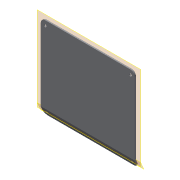
# Autodesk Inventor part: 03_Lid
Saved by Autodesk Inventor 2019.4 (Build 234330000, 330)
## iProperties
Created: 2021-06-05
Part Number: 03_Lid
Material: Generic
Document SubType Name: Modeling
Designer: diederichbenedict
Density: 1 g/cm^3
Appearance: Default
Author: diederichbenedict
Autodesk Inventor part; units mm, degrees
ref_plane "YZ Plane" through (0, 0, 0) normal (1, 0, 0) x (0, 1, 0)
ref_plane "XZ Plane" through (0, 0, 0) normal (0, 1, 0) x (-1, 0, 0)
ref_plane "XY Plane" through (0, 0, 0) normal (0, 0, 1) x (1, 0, 0)
ref_plane "Work Plane1" through (0, 0, 0) normal (0, 0, 1) x (1, 0, 0)
sketch "Sketch1" plane through (0, 0, 0) normal (0, 0, 1) x (1, 0, 0)
  ellipse E0 centre (-7.5, -84.2405) end of major axis (-7.5, -80.461) minor radius 1.5 projected
  ellipse E1 centre (-100.5, -84.2405) end of major axis (-100.5, -80.461) minor radius 1.5 projected
  ellipse E2 centre (-103, -7.7709) end of major axis (-103, -9.3506) minor radius 1.45 projected
  line L0 (-3, -61.2439) -> (-3, -12.7635) projected
  line L1 (-3, -61.2439) -> (-18, -61.2439) projected
  line L2 (-18, -90.5398) -> (-18, -61.2439) projected
  line L3 (0, -90.5398) -> (-18, -90.5398) projected
  line L4 (0, -7.7709) -> (0, -90.5398) projected
  ellipse E3 centre (-5, -7.7709) end of major axis (-5, -13.2183) minor radius 5 (0, -7.7709) -> (-5, -2.3235) ccw projected
  line L5 (-103, -2.3235) -> (-5, -2.3235) projected
  ellipse E4 centre (-103, -7.7709) end of major axis (-103, -13.2183) minor radius 5 (-103, -2.3235) -> (-108, -7.7709) ccw projected
  line L6 (-108, -90.5398) -> (-108, -7.7709) projected
  line L7 (-95, -90.5398) -> (-108, -90.5398) projected
  line L8 (-95, -61.2439) -> (-95, -90.5398) projected
  line L9 (-105, -61.2439) -> (-95, -61.2439) projected
  line L10 (-105, -12.7635) -> (-105, -61.2439) projected
  ellipse E5 centre (-103, -7.7709) end of major axis (-103, -13.2183) minor radius 5 (-105, -12.7635) -> (-98.4174, -5.5919) ccw projected
  line L11 (-9.5826, -5.5919) -> (-98.4174, -5.5919) projected
  ellipse E6 centre (-5, -7.7709) end of major axis (-5, -13.2183) minor radius 5 (-9.5826, -5.5919) -> (-3, -12.7635) ccw projected
  ellipse E7 centre (-5, -7.7709) end of major axis (-5, -9.3506) minor radius 1.45 projected
  line L12 (-18, -90.5398) -> (-95, -90.5398)
  point P0 (0, 0)
  constraints: 2 end point, 1 horizontal, 8 other
extrude "Extrusion1" add sketch "Sketch1" along normal blind 1.5 contours E0 | E1 | L1 L2 L12 L8 L9 L10 E5 L11 E6 L0 | L0 E6 L11 E5 L10 L9 L8 L7 L6 E4 L5 E3 L4 L3 L2 L1
ref_plane "Work Plane2" through (-54, -57.5226, 14.2761) normal (0, -0.3968725, 0.9178738) x (1, 0, 0)
sketch "Sketch2" plane through (-54, -57.5226, 14.2761) normal (0, -0.3968725, 0.9178738) x (1, 0, 0)
  circle A0 centre (49, -40) radius 1.45 projected
  circle A1 centre (-49, -40) radius 1.45 projected
  line L0 (-41, -35.9714) -> (-54, -35.9714) projected
  line L1 (-54, -40) -> (-54, -35.9714) projected
  arc A2 (-54, -40) -> (-49, -45) centre (-49, -40) ccw projected
  line L2 (49, -45) -> (-49, -45) projected
  arc A3 (49, -45) -> (54, -40) centre (49, -40) ccw projected
  line L3 (54, -35.9714) -> (54, -40) projected
  line L4 (54, -35.9714) -> (36, -35.9714) projected
  line L5 (36, -42) -> (36, -35.9714) projected
  line L6 (-41, -42) -> (36, -42) projected
  line L7 (-41, -35.9714) -> (-41, -42) projected
  line L8 (36, -35.9714) -> (-41, -35.9714)
  line L9 (-54, -35.9714) -> (54, -35.9714) projected
  line L10 (-54, 40) -> (-54, -35.9714) projected
  line L11 (54, -35.3761) -> (54, 40.5953) projected
  line L12 (-54, -35.9714) -> (54, -35.9714)
  line L13 (54, -35.9714) -> (54, -35.3761)
  line L14 (54, -35.3761) -> (-54, -35.3761)
  line L15 (-54, -35.3761) -> (-54, -35.9714)
  point P0 (54, 47.1327)
  constraints: 10 end point, 2 parallel, 1 collinear, 1 horizontal, 1 perpendicular
extrude "Extrusion2" add sketch "Sketch2" along normal up to surface (1.3768 mm away)
sketch "Sketch3" plane through (0, 0, 1.5) normal (0, 0, 1) x (1, 0, 0)
  ellipse E0 centre (-5, -7.7709) end of major axis (-5, -6.1911) minor radius 1.45 projected
  ellipse E1 centre (-103, -7.7709) end of major axis (-103, -6.1911) minor radius 1.45 projected
  line L0 (-108, -90.5398) -> (0, -90.5398) projected
  line L1 (0, -90.5398) -> (0, -7.7709) projected
  ellipse E2 centre (-5, -7.7709) end of major axis (-5, -13.2183) minor radius 5 (0, -7.7709) -> (-5, -2.3235) ccw projected
  line L2 (-5, -2.3235) -> (-103, -2.3235) projected
  ellipse E3 centre (-103, -7.7709) end of major axis (-103, -13.2183) minor radius 5 (-103, -2.3235) -> (-108, -7.7709) ccw projected
  line L3 (-108, -7.7709) -> (-108, -90.5398) projected
  line L4 (-3.7152, -59.4836) -> (-104.3916, -59.4836) construction
  line L5 (-104.3916, -59.4836) -> (-104.3916, -42.5544) construction
  line L6 (-104.3916, -42.5544) -> (-3.7152, -42.5544) construction
  line L7 (-3.7152, -42.5544) -> (-3.7152, -59.4836) construction
  spline S0 degree 2 poles (-14.2682, -57.7177) (-15.0084, -56.8506) (-15.8332, -54.3128) (-15.8332, -52.6844) knots 0 0 0 1 2 2 2
  spline S1 degree 2 poles (-15.8332, -52.6844) (-15.8332, -51.0983) (-15.0296, -48.5288) (-14.2682, -47.6617) knots 0 0 0 1 2 2 2
  spline S2 degree 2 poles (-14.2682, -47.6617) (-13.4646, -46.7523) (-11.3392, -45.8852) (-10.0597, -45.8852) knots 0 0 0 1 2 2 2
  spline S3 degree 2 poles (-10.0597, -45.8852) (-8.7379, -45.8852) (-6.6231, -46.784) (-5.8512, -47.6617) knots 0 0 0 1 2 2 2
  spline S4 degree 2 poles (-5.8512, -47.6617) (-5.1004, -48.5288) (-4.2968, -51.0771) (-4.2968, -52.6844) knots 0 0 0 1 2 2 2
  spline S5 degree 2 poles (-4.2968, -52.6844) (-4.2968, -54.3234) (-5.111, -56.8189) (-5.8618, -57.7177) knots 0 0 0 1 2 2 2
  spline S6 degree 2 poles (-5.8618, -57.7177) (-6.6231, -58.5848) (-8.7485, -59.4836) (-10.0597, -59.4836) knots 0 0 0 1 2 2 2
  spline S7 degree 2 poles (-10.0597, -59.4836) (-11.392, -59.4836) (-13.528, -58.553) (-14.2682, -57.7177) knots 0 0 0 1 2 2 2
  spline S8 degree 2 poles (-14.025, -52.6844) (-14.025, -53.9744) (-13.4646, -55.9729) (-12.957, -56.6285) knots 0 0 0 1 2 2 2
  spline S9 degree 2 poles (-12.957, -56.6285) (-12.4389, -57.3053) (-10.9797, -57.982) (-10.0703, -57.982) knots 0 0 0 1 2 2 2
  spline S10 degree 2 poles (-10.0703, -57.982) (-9.1292, -57.982) (-7.7122, -57.3264) (-7.173, -56.6285) knots 0 0 0 1 2 2 2
  spline S11 degree 2 poles (-7.173, -56.6285) (-6.6548, -55.9624) (-6.105, -53.9533) (-6.105, -52.6844) knots 0 0 0 1 2 2 2
  spline S12 degree 2 poles (-6.105, -52.6844) (-6.105, -50.1149) (-8.2621, -47.3867) (-10.0703, -47.3867) knots 0 0 0 1 2 2 2
  spline S13 degree 2 poles (-10.0703, -47.3867) (-11.8785, -47.3867) (-14.025, -50.1149) (-14.025, -52.6844) knots 0 0 0 1 2 2 2
  line L8 (-25.4134, -46.1601) -> (-17.3664, -46.1601)
  line L9 (-17.3664, -46.1601) -> (-17.3664, -48.0106)
  spline S14 degree 2 poles (-17.3664, -48.0106) (-18.2335, -48.8248) (-19.7773, -50.3369) (-20.5175, -51.1511) knots 0 0 0 1 2 2 2
  spline S15 degree 2 poles (-20.5175, -51.1511) (-22.0085, -52.7901) (-23.0976, -54.7569) (-23.0976, -55.8038) knots 0 0 0 1 2 2 2
  spline S16 degree 2 poles (-23.0976, -55.8038) (-23.0976, -56.3536) (-22.7592, -57.1784) (-22.4526, -57.4428) knots 0 0 0 1 2 2 2
  spline S17 degree 2 poles (-22.4526, -57.4428) (-22.1459, -57.7071) (-21.3423, -57.9715) (-20.8559, -57.9715) knots 0 0 0 1 2 2 2
  spline S18 degree 2 poles (-20.8559, -57.9715) (-20.3906, -57.9715) (-19.439, -57.7388) (-19.0054, -57.5591) knots 0 0 0 1 2 2 2
  spline S19 degree 2 poles (-19.0054, -57.5591) (-18.6353, -57.411) (-17.948, -56.9881) (-17.7365, -56.84) knots 0 0 0 1 2 2 2
  line L10 (-17.7365, -56.84) -> (-17.6414, -56.84)
  line L11 (-17.6414, -56.84) -> (-17.6414, -58.7011)
  spline S20 degree 2 poles (-17.6414, -58.7011) (-18.1806, -58.9654) (-20.1157, -59.4836) (-20.9828, -59.4836) knots 0 0 0 1 2 2 2
  spline S21 degree 2 poles (-20.9828, -59.4836) (-22.8121, -59.4836) (-24.8741, -57.5485) (-24.8741, -55.8989) knots 0 0 0 1 2 2 2
  spline S22 degree 2 poles (-24.8741, -55.8989) (-24.8741, -55.127) (-24.5146, -53.837) (-24.1973, -53.2871) knots 0 0 0 1 2 2 2
  spline S23 degree 2 poles (-24.1973, -53.2871) (-23.8801, -52.7161) (-22.9602, -51.5953) (-22.4526, -51.056) knots 0 0 0 1 2 2 2
  spline S24 degree 2 poles (-22.4526, -51.056) (-21.6278, -50.1572) (-19.6082, -48.2327) (-19.0054, -47.6722) knots 0 0 0 1 2 2 2
  line L12 (-19.0054, -47.6722) -> (-25.4134, -47.6722)
  line L13 (-25.4134, -47.6722) -> (-25.4134, -46.1601)
  spline S25 degree 2 poles (-42.3637, -57.7177) (-43.1039, -56.8506) (-43.9287, -54.3128) (-43.9287, -52.6844) knots 0 0 0 1 2 2 2
  spline S26 degree 2 poles (-43.9287, -52.6844) (-43.9287, -51.0983) (-43.125, -48.5288) (-42.3637, -47.6617) knots 0 0 0 1 2 2 2
  spline S27 degree 2 poles (-42.3637, -47.6617) (-41.5601, -46.7523) (-39.4347, -45.8852) (-38.1552, -45.8852) knots 0 0 0 1 2 2 2
  spline S28 degree 2 poles (-38.1552, -45.8852) (-36.8334, -45.8852) (-34.7186, -46.784) (-33.9467, -47.6617) knots 0 0 0 1 2 2 2
  spline S29 degree 2 poles (-33.9467, -47.6617) (-33.1959, -48.5288) (-32.3923, -51.0771) (-32.3923, -52.6844) knots 0 0 0 1 2 2 2
  spline S30 degree 2 poles (-32.3923, -52.6844) (-32.3923, -54.3234) (-33.2065, -56.8189) (-33.9573, -57.7177) knots 0 0 0 1 2 2 2
  spline S31 degree 2 poles (-33.9573, -57.7177) (-34.7186, -58.5848) (-36.844, -59.4836) (-38.1552, -59.4836) knots 0 0 0 1 2 2 2
  spline S32 degree 2 poles (-38.1552, -59.4836) (-39.4875, -59.4836) (-41.6235, -58.553) (-42.3637, -57.7177) knots 0 0 0 1 2 2 2
  spline S33 degree 2 poles (-42.1205, -52.6844) (-42.1205, -53.9744) (-41.5601, -55.9729) (-41.0525, -56.6285) knots 0 0 0 1 2 2 2
  spline S34 degree 2 poles (-41.0525, -56.6285) (-40.5344, -57.3053) (-39.0751, -57.982) (-38.1658, -57.982) knots 0 0 0 1 2 2 2
  spline S35 degree 2 poles (-38.1658, -57.982) (-37.2247, -57.982) (-35.8077, -57.3264) (-35.2685, -56.6285) knots 0 0 0 1 2 2 2
  spline S36 degree 2 poles (-35.2685, -56.6285) (-34.7503, -55.9624) (-34.2005, -53.9533) (-34.2005, -52.6844) knots 0 0 0 1 2 2 2
  spline S37 degree 2 poles (-34.2005, -52.6844) (-34.2005, -50.1149) (-36.3576, -47.3867) (-38.1658, -47.3867) knots 0 0 0 1 2 2 2
  spline S38 degree 2 poles (-38.1658, -47.3867) (-39.9739, -47.3867) (-42.1205, -50.1149) (-42.1205, -52.6844) knots 0 0 0 1 2 2 2
  spline S39 degree 2 poles (-53.9107, -51.3203) (-53.9107, -48.8671) (-51.5738, -45.9698) (-49.7868, -45.9698) knots 0 0 0 1 2 2 2
  spline S40 degree 2 poles (-49.7868, -45.9698) (-49.0571, -45.9698) (-47.9363, -46.3082) (-47.3547, -46.6571) knots 0 0 0 1 2 2 2
  line L14 (-47.3547, -46.6571) -> (-47.3547, -42.5544)
  line L15 (-47.3547, -42.5544) -> (-45.7051, -42.5544)
  line L16 (-45.7051, -42.5544) -> (-45.7051, -55.9518)
  line L17 (-45.7051, -55.9518) -> (-47.3547, -55.9518)
  line L18 (-47.3547, -55.9518) -> (-47.3547, -54.9261)
  spline S41 degree 2 poles (-47.3547, -54.9261) (-47.968, -55.4865) (-49.4695, -56.2267) (-50.3472, -56.2267) knots 0 0 0 1 2 2 2
  spline S42 degree 2 poles (-50.3472, -56.2267) (-52.0285, -56.2267) (-53.9107, -53.562) (-53.9107, -51.3203) knots 0 0 0 1 2 2 2
  spline S43 degree 2 poles (-52.2082, -51.13) (-52.2082, -52.8113) (-51.1402, -54.6618) (-49.9454, -54.6618) knots 0 0 0 1 2 2 2
  spline S44 degree 2 poles (-49.9454, -54.6618) (-49.2475, -54.6618) (-47.9363, -54.0379) (-47.3547, -53.5515) knots 0 0 0 1 2 2 2
  line L19 (-47.3547, -53.5515) -> (-47.3547, -47.9895)
  spline S45 degree 2 poles (-47.3547, -47.9895) (-47.9997, -47.6828) (-48.9197, -47.4502) (-49.5118, -47.4502) knots 0 0 0 1 2 2 2
  spline S46 degree 2 poles (-49.5118, -47.4502) (-50.7913, -47.4502) (-52.2082, -49.3324) (-52.2082, -51.13) knots 0 0 0 1 2 2 2
  spline S47 degree 2 poles (-59.8745, -45.9381) (-57.527, -45.9381) (-54.9469, -48.571) (-54.9469, -51.0031) knots 0 0 0 1 2 2 2
  spline S48 degree 2 poles (-54.9469, -51.0031) (-54.9469, -53.3929) (-57.453, -56.2267) (-59.4727, -56.2267) knots 0 0 0 1 2 2 2
  spline S49 degree 2 poles (-59.4727, -56.2267) (-60.382, -56.2267) (-61.7884, -55.698) (-62.3065, -55.1376) knots 0 0 0 1 2 2 2
  spline S50 degree 2 poles (-62.3065, -55.1376) (-62.8352, -54.5772) (-63.3957, -52.9593) (-63.3957, -51.7856) knots 0 0 0 1 2 2 2
  line L20 (-63.3957, -51.7856) -> (-63.3957, -50.8868)
  line L21 (-63.3957, -50.8868) -> (-56.6176, -50.8868)
  spline S51 degree 2 poles (-56.6176, -50.8868) (-56.6176, -49.1843) (-58.3307, -47.3762) (-59.8533, -47.3762) knots 0 0 0 1 2 2 2
  spline S52 degree 2 poles (-59.8533, -47.3762) (-60.3926, -47.3762) (-61.4395, -47.6194) (-61.8624, -47.8097) knots 0 0 0 1 2 2 2
  spline S53 degree 2 poles (-61.8624, -47.8097) (-62.3065, -48.0212) (-62.9198, -48.3913) (-63.1207, -48.5605) knots 0 0 0 1 2 2 2
  line L22 (-63.1207, -48.5605) -> (-63.2159, -48.5605)
  line L23 (-63.2159, -48.5605) -> (-63.2159, -46.7629)
  spline S54 degree 2 poles (-63.2159, -46.7629) (-62.9304, -46.6466) (-62.0633, -46.3082) (-61.725, -46.213) knots 0 0 0 1 2 2 2
  spline S55 degree 2 poles (-61.725, -46.213) (-61.2491, -46.0756) (-60.4666, -45.9381) (-59.8745, -45.9381) knots 0 0 0 1 2 2 2
  spline S56 degree 2 poles (-61.7884, -52.1451) (-61.7673, -52.8113) (-61.4923, -53.7841) (-61.228, -54.1119) knots 0 0 0 1 2 2 2
  spline S57 degree 2 poles (-61.228, -54.1119) (-60.9425, -54.482) (-60.0437, -54.8732) (-59.3775, -54.8732) knots 0 0 0 1 2 2 2
  spline S58 degree 2 poles (-59.3775, -54.8732) (-58.7219, -54.8732) (-57.8019, -54.482) (-57.4213, -54.1013) knots 0 0 0 1 2 2 2
  spline S59 degree 2 poles (-57.4213, -54.1013) (-57.0512, -53.7101) (-56.6705, -52.769) (-56.6176, -52.1451) knots 0 0 0 1 2 2 2
  line L24 (-56.6176, -52.1451) -> (-61.7884, -52.1451)
  line L25 (-72.7538, -46.1601) -> (-71.1042, -46.1601)
  line L26 (-71.1042, -46.1601) -> (-71.1042, -51.7433)
  spline S60 degree 2 poles (-71.1042, -51.7433) (-71.1042, -52.42) (-70.9773, -53.5832) (-70.787, -53.9321) knots 0 0 0 1 2 2 2
  spline S61 degree 2 poles (-70.787, -53.9321) (-70.5861, -54.3022) (-69.867, -54.6618) (-69.2537, -54.6618) knots 0 0 0 1 2 2 2
  spline S62 degree 2 poles (-69.2537, -54.6618) (-68.6404, -54.6618) (-67.3398, -54.0062) (-66.7159, -53.4775) knots 0 0 0 1 2 2 2
  line L27 (-66.7159, -53.4775) -> (-66.7159, -46.1601)
  line L28 (-66.7159, -46.1601) -> (-65.0664, -46.1601)
  line L29 (-65.0664, -46.1601) -> (-65.0664, -55.9518)
  line L30 (-65.0664, -55.9518) -> (-66.7159, -55.9518)
  line L31 (-66.7159, -55.9518) -> (-66.7159, -54.8627)
  spline S63 degree 2 poles (-66.7159, -54.8627) (-67.4561, -55.5288) (-68.8836, -56.2267) (-69.6873, -56.2267) knots 0 0 0 1 2 2 2
  spline S64 degree 2 poles (-69.6873, -56.2267) (-71.1254, -56.2267) (-72.7538, -54.3234) (-72.7538, -52.5152) knots 0 0 0 1 2 2 2
  line L32 (-72.7538, -52.5152) -> (-72.7538, -46.1601)
  spline S65 degree 2 poles (-84.4276, -57.7177) (-85.1678, -56.8506) (-85.9926, -54.3128) (-85.9926, -52.6844) knots 0 0 0 1 2 2 2
  spline S66 degree 2 poles (-85.9926, -52.6844) (-85.9926, -51.0983) (-85.189, -48.5288) (-84.4276, -47.6617) knots 0 0 0 1 2 2 2
  spline S67 degree 2 poles (-84.4276, -47.6617) (-83.624, -46.7523) (-81.4986, -45.8852) (-80.2191, -45.8852) knots 0 0 0 1 2 2 2
  spline S68 degree 2 poles (-80.2191, -45.8852) (-78.8974, -45.8852) (-76.7825, -46.784) (-76.0106, -47.6617) knots 0 0 0 1 2 2 2
  spline S69 degree 2 poles (-76.0106, -47.6617) (-75.2599, -48.5288) (-74.4562, -51.0771) (-74.4562, -52.6844) knots 0 0 0 1 2 2 2
  spline S70 degree 2 poles (-74.4562, -52.6844) (-74.4562, -54.3234) (-75.2704, -56.8189) (-76.0212, -57.7177) knots 0 0 0 1 2 2 2
  spline S71 degree 2 poles (-76.0212, -57.7177) (-76.7825, -58.5848) (-78.9079, -59.4836) (-80.2191, -59.4836) knots 0 0 0 1 2 2 2
  spline S72 degree 2 poles (-80.2191, -59.4836) (-81.5515, -59.4836) (-83.6874, -58.553) (-84.4276, -57.7177) knots 0 0 0 1 2 2 2
  spline S73 degree 2 poles (-84.1844, -52.6844) (-84.1844, -53.9744) (-83.624, -55.9729) (-83.1164, -56.6285) knots 0 0 0 1 2 2 2
  spline S74 degree 2 poles (-83.1164, -56.6285) (-82.5983, -57.3053) (-81.1391, -57.982) (-80.2297, -57.982) knots 0 0 0 1 2 2 2
  spline S75 degree 2 poles (-80.2297, -57.982) (-79.2886, -57.982) (-77.8717, -57.3264) (-77.3324, -56.6285) knots 0 0 0 1 2 2 2
  spline S76 degree 2 poles (-77.3324, -56.6285) (-76.8143, -55.9624) (-76.2644, -53.9533) (-76.2644, -52.6844) knots 0 0 0 1 2 2 2
  spline S77 degree 2 poles (-76.2644, -52.6844) (-76.2644, -50.1149) (-78.4215, -47.3867) (-80.2297, -47.3867) knots 0 0 0 1 2 2 2
  spline S78 degree 2 poles (-80.2297, -47.3867) (-82.0379, -47.3867) (-84.1844, -50.1149) (-84.1844, -52.6844) knots 0 0 0 1 2 2 2
  line L33 (-95.3719, -46.1601) -> (-93.3522, -46.1601)
  line L34 (-93.3522, -46.1601) -> (-90.973, -49.8399)
  line L35 (-90.973, -49.8399) -> (-88.5304, -46.1601)
  line L36 (-88.5304, -46.1601) -> (-86.6588, -46.1601)
  line L37 (-86.6588, -46.1601) -> (-90.0531, -51.0137)
  line L38 (-90.0531, -51.0137) -> (-86.6905, -55.9518)
  line L39 (-86.6905, -55.9518) -> (-88.7102, -55.9518)
  line L40 (-88.7102, -55.9518) -> (-91.0788, -52.3037)
  line L41 (-91.0788, -52.3037) -> (-93.5002, -55.9518)
  line L42 (-93.5002, -55.9518) -> (-95.3719, -55.9518)
  line L43 (-95.3719, -55.9518) -> (-91.9987, -51.1194)
  line L44 (-91.9987, -51.1194) -> (-95.3719, -46.1601)
  line L45 (-104.3387, -55.9518) -> (-99.0728, -42.5544)
  line L46 (-99.0728, -42.5544) -> (-97.3069, -42.5544)
  line L47 (-97.3069, -42.5544) -> (-99.0622, -46.636)
  line L48 (-99.0622, -46.636) -> (-95.5093, -55.9518)
  line L49 (-95.5093, -55.9518) -> (-97.2858, -55.9518)
  line L50 (-97.2858, -55.9518) -> (-99.961, -48.6979)
  line L51 (-99.961, -48.6979) -> (-102.6257, -55.9518)
  line L52 (-102.6257, -55.9518) -> (-104.3387, -55.9518)
  point P0 (0, 0)
  constraints: 6 other
extrude "Extrusion3" cut sketch "Sketch3" against normal blind 0.5 contours S0 S1 S2 S3 S4 S5 S6 S7 | L8 L9 S14 S15 S16 S17 S18 S19 L10 L11 S20 S21 S22 S23 S24 L12 L13 | S25 S26 S27 S28 S29 S30 S31 S32 | S39 S40 L14 L15 L16 L17 L18 S41 S42 | S47 S48 S49 S50 L20 L21 S51 S52 S53 L22 L23 S54 S55 | L25 L26 S60 S61 S62 L27 L28 L29 L30 L31 S63 S64 L32 | S65 S66 S67 S68 S69 S70 S71 S72 | L33 L34 L35 L36 L37 L38 L39 L40 L41 L42 L43 L44 | L45 L46 L47 L48 L49 L50 L51 L52
body "Solid1"
